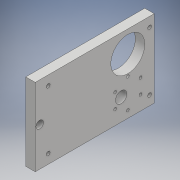
# Autodesk Inventor part: paroismoteur
Saved by Autodesk Inventor 2017 SP1 (Build 210196100, 196)
## iProperties
Part Number: paroismoteur
Material: Générique
Document SubType Name: Modeling
Designer: Sylvain
Density: 1 g/cm^3
Appearance: Par défaut
Author: Sylvain
Autodesk Inventor part; units mm, degrees
ref_plane "YZ Plane" through (0, 0, 0) normal (1, 0, 0) x (0, 1, 0)
ref_plane "XZ Plane" through (0, 0, 0) normal (0, 1, 0) x (-1, 0, 0)
ref_plane "XY Plane" through (0, 0, 0) normal (0, 0, 1) x (1, 0, 0)
sketch "Esquisse1" plane through (0, 0, 0) normal (1, 0, 0) x (0, 1, 0)
  line L0 (0, 0) -> (-126, 0)
  line L1 (-126, -82) -> (0, -82)
  circle A0 centre (-23, -23) radius 18
  circle A1 centre (-23, -59) radius 18
  circle A2 centre (-116.2792, -41) radius 4
  line L2 (-120.2792, 0) -> (-120.2792, -82)
  circle A3 centre (-30, -59) radius 6
  circle A4 centre (-23, -43.5) radius 1.5
  circle A5 centre (-23, -74.5) radius 1.5
  circle A6 centre (-9.5766, -51.25) radius 1.5
  circle A7 centre (-9.5766, -66.75) radius 1.5
  line L3 (-23, -59) -> (-30, -59)
  line L4 (-23, -59) -> (-23, -43.5)
  line L5 (-23, -59) -> (-23, -74.5)
  circle A8 centre (-36.4234, -51.25) radius 1.5
  circle A9 centre (-36.4234, -66.75) radius 1.5
  line L6 (0, -82) -> (5, -82)
  line L7 (5, -82) -> (5, 0)
  line L8 (5, 0) -> (0, 0)
  line L9 (-5, -82) -> (-5, 0)
  line L10 (0, -72) -> (0, -10)
  circle A10 centre (0, -72) radius 2
  circle A11 centre (0, -10) radius 2
  line L11 (5, 0) -> (0, 0)
  line L12 (5, -82) -> (-5, -82)
  line L13 (-107.2792, -10) -> (-107.2792, -72)
  circle A12 centre (-107.2792, -10) radius 2
  circle A13 centre (-107.2792, -72) radius 2
  line L14 (-120.2792, 0) -> (-126, 0)
  line L15 (-126, 0) -> (-126, -82)
  line L16 (-126, -82) -> (-120.2792, -82)
  line L17 (-120.2792, -82) -> (-120.2792, 0)
  dimension "d0" = 82
  dimension "d2" = 36
  dimension "d3" = 23
  dimension "d4" = 36
  dimension "d5" = 23
  dimension "d6" = 8
  dimension "d7" = 95
  dimension "d8" = 41
  dimension "d12" = 4
  dimension "d13" = 12
  dimension "d14" = 7
  dimension "d15" = 3
  dimension "d16" = 15.5
  dimension "d17" = 3
  dimension "d18" = 15.5
  dimension "d19" = 3
  dimension "d20" = 3
  dimension "d21" = 60
  dimension "d22" = 60
  dimension "d23" = 15.5
  dimension "d25" = 0
  dimension "d26" = 15.5
  dimension "d27" = 3
  dimension "d28" = 3
  dimension "d29" = 15.5
  dimension "d30" = 15.5
  dimension "d31" = 60
  dimension "d32" = 60
  dimension "d38" = 82
  dimension "d39" = 28
  dimension "d40" = 10
  dimension "d41" = 5
  dimension "d42" = 62
  dimension "d43" = 10
  dimension "d44" = 4
  dimension "d45" = 4
  dimension "d46" = 5
  dimension "d47" = 82
  dimension "d48" = 10
  dimension "d49" = 28
  dimension "d61" = 62
  dimension "d62" = 13
  dimension "d63" = 10
  dimension "d64" = 4
  dimension "d65" = 4
  dimension "d76" = 126
  dimension "d77" = 126
  constraints: 36 end point, 14 centre point, 6 coincident, 5 parallel, 4 horizontal, 4 perpendicular, 4 point on line, 3 vertical, 2 collinear
  measures "d0" distance of L1.end L0.start
  measures "d2" diameter of A0
  measures "d3" distance from line of L0 A0.centre
  measures "d4" diameter of A1
  measures "d5" distance from line of L1 L3.start
  measures "d6" diameter of A2
  measures "d7" distance of A2.centre A0.centre
  measures "d8" distance from line of L0 A2.centre
  measures "d12" distance from line of L2 A2.centre
  measures "d13" diameter of A3
  measures "d14" distance of L3.end L3.start
  measures "d15" diameter of A4
  measures "d16" distance of L3.start L4.end
  measures "d17" diameter of A5
  measures "d18" distance of L3.start L5.end
  measures "d19" diameter of A6
  measures "d20" diameter of A7
  measures "d23" distance of L3.start A6.centre
  measures "d25" distance from line of point (0, 0) L0
  measures "d26" distance of L3.start A7.centre
  measures "d27" diameter of A8
  measures "d28" diameter of A9
  measures "d29" distance of A8.centre L3.start
  measures "d30" distance of A9.centre L3.start
  measures "d38" distance between parallel lines of L8 L6
  measures "d39" distance from line of A0.centre L7
  measures "d40" distance between parallel lines of L9 L7
  measures "d41" distance between parallel lines of L7 L10
  measures "d42" distance of L10.start L10.end
  measures "d43" distance of L1.end L10.start
  measures "d44" diameter of A10
  measures "d45" diameter of A11
  measures "d46" distance from line of point (0, 0) L7
  measures "d47" distance between parallel lines of L0 L1
  measures "d48" distance of point (0, 0) point (0, -10)
  measures "d49" distance from line of L3.start L7
  measures "d61" distance of L13.start L13.end
  measures "d62" distance between parallel lines of L2 L13
  measures "d63" distance from line of L0 L13.start
  measures "d64" diameter of A12
  measures "d65" diameter of A13
  measures "d76" distance of L0.start L0.end
  measures "d77" distance of L1.start L1.end
extrude "Extrusion1" add sketch "Esquisse1" along normal blind 10 contours L9 A0 A1 L1 L2 L0 | L9 A1 A0 | A1 | A13 | A12
sketch "Esquisse2" plane through (10, -23, -23) normal (1, 0, 0) x (0, 0, -1)
  line L0 (0, 18) -> (-23, 18) projected
  line L1 (-23, 18) -> (59, 18)
  line L2 (59, 18) -> (59, 28)
  line L3 (59, 28) -> (-23, 28)
  line L4 (-23, 28) -> (-23, 18)
  line L5 (-13, 23) -> (49, 23)
  circle A0 centre (-13, 23) radius 2
  circle A1 centre (49, 23) radius 2
  point P0 (-23, 23)
  dimension "d52" = 82
  dimension "d53" = 10
  dimension "d54" = 62
  dimension "d55" = 10
  dimension "d56" = 4
  dimension "d57" = 4
  dimension "d58" = 5
  constraints: 10 end point, 2 centre point, 2 coincident, 2 horizontal, 2 parallel, 1 perpendicular
  measures "d52" distance between parallel lines of L2 L4
  measures "d53" distance between parallel lines of L1 L3
  measures "d54" distance of L5.start L5.end
  measures "d55" distance from line of L5.start L4
  measures "d56" diameter of A0
  measures "d57" diameter of A1
  measures "d58" distance between parallel lines of L3 L5
extrude "Extrusion2" add sketch "Esquisse2" against normal blind 10
sketch "Esquisse3" plane through (10, -116.2792, -41) normal (1, 0, 0) x (0, 0, -1)
  line L0 (-31, 9) -> (31, 9)
  line L1 (-41, 121.2792) -> (-41, -4) projected
  line L2 (-41, -4) -> (0, -4) projected
  point P0 (-41, 116.2792)
  dimension "d66" = 62
  dimension "d67" = 10
  dimension "d68" = 13
  constraints: 2 coincident, 2 end point, 1 horizontal
  measures "d66" distance of L0.start L0.end
  measures "d67" distance from line of L1 L0.start
  measures "d68" distance between parallel lines of L2 L0
hole "Perçage1" at (10, -107.2792, -10) at (10, -107.2792, -72) direction (-1, 0, 0) diameter 4 end through all
sketch "Esquisse4" plane through (0, -120.2792, -41) normal (0, -1, 0) x (1, 0, 0)
  line L0 (0, 0) -> (0, -41) projected
  line L1 (10, 41) -> (0, 41)
  line L2 (0, 41) -> (0, -41)
  line L3 (0, -41) -> (10, -41)
  line L4 (10, -41) -> (10, 41)
  dimension "d78" = 10
  dimension "d79" = 82
  constraints: 8 end point, 2 parallel, 1 horizontal, 1 perpendicular
  measures "d78" distance of L1.start L1.end
  measures "d79" distance of L3.end L1.start
extrude "Extrusion3" add sketch "Esquisse4" along normal blind 0.72
